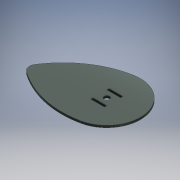
# Autodesk Inventor part: leva00
Saved by Autodesk Inventor 2016 (Build 200138000, 138)
## iProperties
Created: 2016-09-20
Part Number: leva00
Material: Madera (abedul)
Document SubType Name: Modeling
Designer: i95sa
Density: 0.55 g/cm^3
Appearance: Gris plomo - Pulido
Author: i95sa
Autodesk Inventor part; units mm, degrees
ref_plane "YZ Plane" through (0, 0, 0) normal (1, 0, 0) x (0, 1, 0)
ref_plane "XZ Plane" through (0, 0, 0) normal (0, 1, 0) x (-1, 0, 0)
ref_plane "XY Plane" through (0, 0, 0) normal (0, 0, 1) x (1, 0, 0)
sketch "Boceto1" plane through (0, 0, 0) normal (0, 0, 1) x (1, 0, 0)
  arc A0 (59.8262, 11.4125) -> (-59.8262, -11.4125) centre (0, 0) ccw
  arc A1 (-92.0678, -17.5629) -> (-119.6799, -22.8302) centre (-105.8739, -20.1965) ccw
  line L0 (-123.6771, -23.5927) -> (-126.3108, -9.7866)
  line L1 (-10.703, 59.9572) -> (-15.0924, 82.9673)
  line L2 (-15.0924, 82.9673) -> (-126.3108, -9.7866)
  line L3 (-126.3108, -9.7866) -> (-83.1351, 26.221)
  arc A2 (-10.703, 59.9572) -> (-83.1351, 26.221) centre (16.6855, -93.4708) ccw
  arc A3 (-83.1351, 26.221) -> (-117.6306, -12.4945) centre (29.5849, -108.9381) ccw
  line L4 (4.602, 0.8779) -> (59.8262, 11.4125)
  line L5 (-4.602, -0.8779) -> (-123.6771, -23.5927)
  arc A4 (-59.8262, -11.4125) -> (59.8262, 11.4125) centre (0, 0) ccw
  arc A5 (-119.6799, -22.8302) -> (-92.0678, -17.5629) centre (-105.8739, -20.1965) ccw
  line L6 (-123.6771, -23.5927) -> (-121.0435, -37.3987)
  line L7 (12.1203, -59.6868) -> (16.5098, -82.6969)
  line L8 (16.5098, -82.6969) -> (-121.0435, -37.3987)
  line L9 (-121.0435, -37.3987) -> (-67.6445, -54.9838)
  arc A6 (-67.6445, -54.9838) -> (12.1203, -59.6868) centre (-18.8951, 93.0493) ccw
  arc A7 (-113.9697, -31.6857) -> (-67.6445, -54.9838) centre (-12.5954, 112.1791) ccw
  dimension "d0" = 121.81
  dimension "d6" = 28.11
  dimension "d7" = 14.055
  dimension "d8" = 23.425
  dimension "d9" = 56.22
  constraints: 20 end point, 20 point on circle, 8 centre point, 6 symmetric about line, 5 point on line, 4 tangent, 1 collinear, 4 other
  measures "d0" diameter of A0
  measures "d6" diameter of A1
  measures "d7" distance of L0.start L0.end
  measures "d8" distance of L1.start L1.end
  measures "d9" distance of L0.end L3.end
extrude "Extrusión2" add sketch "Boceto1" along normal blind 4 contours A4 A0 | A0 L5 A1 A3 A2 | A6 A7 A5 L5 A4 | L5 A1 | A5 L5
sketch "Boceto2" plane through (0, 0, 4) normal (0, 0, 1) x (1, 0, 0)
  line L0 (0, 0) -> (0, 12.5)
  line L1 (0, 12.5) -> (-12.5, 12.5)
  line L2 (-12.5, 12.5) -> (-12.5, 16.7)
  line L3 (-12.5, 16.7) -> (12.5, 16.7)
  line L4 (12.5, 16.7) -> (12.5, 12.5)
  line L5 (12.5, 12.5) -> (0, 12.5)
  line L6 (0, 0) -> (12.5, 0)
  line L7 (0, 0) -> (0, -12.5)
  line L8 (0, -12.5) -> (-12.5, -12.5)
  line L9 (-12.5, -12.5) -> (-12.5, -16.7)
  line L10 (-12.5, -16.7) -> (12.5, -16.7)
  line L11 (12.5, -16.7) -> (12.5, -12.5)
  line L12 (12.5, -12.5) -> (0, -12.5)
  circle A0 centre (0, 0) radius 5
  dimension "d24" = 12.5
  dimension "d25" = 12.5
  dimension "d26" = 4.2
  dimension "d27" = 25
  dimension "d28" = 10
  constraints: 26 end point, 5 perpendicular, 5 symmetric about line, 3 point on line, 1 centre point, 1 coincident, 1 parallel, 1 vertical
  measures "d24" distance of L0.start L0.end
  measures "d25" distance of L0.end L1.end
  measures "d26" distance of L1.end L2.end
  measures "d27" distance of L2.end L3.end
  measures "d28" diameter of A0
extrude "Extrusión3" cut sketch "Boceto2" against normal blind 4
